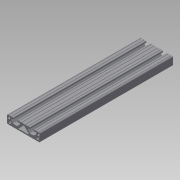
# Autodesk Inventor part: 3034-LITE
Saved by Autodesk Inventor 2013 (Build 170138000, 138)
## iProperties
Created: 2014-04-23
Part Number: 3034-LITE
Material: Generic
Document SubType Name: Modeling
Density: 1 g/cm^3
Vendor: 80/20 Inc.
Engineer: Ross Bowman
Designer: Ross Bowman
Catalog Web Link: 8020.net
Company: 80/20 Inc.
Author: Ross Bowman
Keywords: 80/20 , 8020 , T-Slot , Extrusion
Material: 6105-T5 Aluminum
Autodesk Inventor part; units mm, degrees
ref_plane "YZ Plane" through (0, 0, 0) normal (1, 0, 0) x (0, 1, 0)
ref_plane "XZ Plane" through (0, 0, 0) normal (0, 1, 0) x (-1, 0, 0)
ref_plane "XY Plane" through (0, 0, 0) normal (0, 0, 1) x (1, 0, 0)
sketch "Sketch1" plane through (0, 0, 0) normal (0, 0, 1) x (1, 0, 0)
  circle A0 centre (31.75, -3.175) radius 3.3274
  circle A1 centre (-31.75, -3.175) radius 3.3274
  arc A2 (-30.9118, 7.493) -> (-31.1658, 7.747) centre (-31.1658, 7.493) ccw
  line L0 (-30.9118, 2.5957) -> (-30.9118, 7.493)
  arc A3 (-31.1658, 2.3417) -> (-30.9118, 2.5957) centre (-31.1658, 2.5957) ccw
  line L1 (-36.2712, 2.3417) -> (-31.1658, 2.3417)
  arc A4 (-36.5252, 2.5957) -> (-36.2712, 2.3417) centre (-36.2712, 2.5957) ccw
  line L2 (-36.5252, 4.953) -> (-36.5252, 2.5957)
  arc A5 (-33.7312, 7.747) -> (-36.5252, 4.953) centre (-33.7312, 4.953) ccw
  line L3 (-31.1658, 7.747) -> (-33.7312, 7.747)
  arc A6 (30.9118, 2.5957) -> (31.1658, 2.3417) centre (31.1658, 2.5957) ccw
  line L4 (30.9118, 7.493) -> (30.9118, 2.5957)
  arc A7 (31.1658, 7.747) -> (30.9118, 7.493) centre (31.1658, 7.493) ccw
  line L5 (33.7312, 7.747) -> (31.1658, 7.747)
  arc A8 (36.5252, 4.953) -> (33.7312, 7.747) centre (33.7312, 4.953) ccw
  line L6 (36.5252, 2.5957) -> (36.5252, 4.953)
  arc A9 (36.2712, 2.3417) -> (36.5252, 2.5957) centre (36.2712, 2.5957) ccw
  line L7 (31.1658, 2.3417) -> (36.2712, 2.3417)
  arc A10 (0, 6.0555) -> (-2.3585, 5.1274) centre (-0.1132, 2.8826) ccw
  arc A11 (2.3585, 5.1274) -> (0, 6.0555) centre (0.1132, 2.8826) ccw
  line L8 (11.7359, -4.2517) -> (2.3585, 5.1274)
  arc A12 (10.8378, -6.4196) -> (11.7359, -4.2517) centre (10.8378, -5.1496) ccw
  line L9 (-10.8378, -6.4196) -> (10.8378, -6.4196)
  arc A13 (-11.7359, -4.2517) -> (-10.8378, -6.4196) centre (-10.8378, -5.1496) ccw
  line L10 (-2.3585, 5.1274) -> (-11.7359, -4.2517)
  arc A14 (35.2826, -9.525) -> (38.1, -6.7076) centre (35.2826, -6.7076) ccw
  line L11 (38.1, -6.7076) -> (38.1, 6.7076)
  arc A15 (38.1, 6.7076) -> (35.2826, 9.525) centre (35.2826, 6.7076) ccw
  line L12 (35.2826, 9.525) -> (35.224, 9.525)
  arc A16 (33.7, 9.525) -> (35.224, 9.525) centre (34.462, 9.525) ccw
  line L13 (33.7, 9.525) -> (28.5496, 9.525)
  arc A17 (27.0256, 9.525) -> (28.5496, 9.525) centre (27.7876, 9.525) ccw
  line L14 (27.0256, 9.525) -> (24.7127, 9.525)
  arc A18 (24.7127, 9.525) -> (23.114, 7.9263) centre (24.7127, 7.9263) ccw
  line L15 (23.114, 7.9263) -> (23.114, 7.0358)
  arc A19 (23.114, 7.0358) -> (24.6888, 5.461) centre (24.6888, 7.0358) ccw
  line L16 (24.6888, 5.461) -> (25.8225, 5.461)
  arc A20 (25.8225, 5.461) -> (26.0765, 5.715) centre (25.8225, 5.715) ccw
  line L17 (26.0765, 5.715) -> (26.0765, 5.969)
  arc A21 (26.3305, 6.223) -> (26.0765, 5.969) centre (26.3305, 5.969) ccw
  line L18 (26.3305, 6.223) -> (28.5668, 6.223)
  arc A22 (29.337, 5.4528) -> (28.5668, 6.223) centre (28.5668, 5.4528) ccw
  line L19 (29.337, 5.4528) -> (29.337, 3.4005)
  arc A23 (29.077, 2.7726) -> (29.337, 3.4005) centre (28.4489, 3.4005) ccw
  line L20 (29.077, 2.7726) -> (24.9729, -1.3322)
  arc A24 (21.7509, -2.667) -> (24.9729, -1.3322) centre (21.7509, 1.8892) ccw
  line L21 (21.7509, -2.667) -> (16.4293, -2.667)
  arc A25 (13.0704, -1.2755) -> (16.4293, -2.667) centre (16.4293, 2.0828) ccw
  line L22 (13.0704, -1.2755) -> (9.0233, 2.7723)
  arc A26 (8.763, 3.4008) -> (9.0233, 2.7723) centre (9.6519, 3.4008) ccw
  line L23 (8.763, 3.4008) -> (8.763, 5.4528)
  arc A27 (9.5332, 6.223) -> (8.763, 5.4528) centre (9.5332, 5.4528) ccw
  line L24 (9.5332, 6.223) -> (11.7695, 6.223)
  arc A28 (12.0235, 5.969) -> (11.7695, 6.223) centre (11.7695, 5.969) ccw
  line L25 (12.0235, 5.969) -> (12.0235, 5.715)
  arc A29 (12.0235, 5.715) -> (12.2775, 5.461) centre (12.2775, 5.715) ccw
  line L26 (12.2775, 5.461) -> (13.4112, 5.461)
  arc A30 (13.4112, 5.461) -> (14.986, 7.0358) centre (13.4112, 7.0358) ccw
  line L27 (14.986, 7.0358) -> (14.986, 7.9502)
  arc A31 (14.986, 7.9502) -> (13.4112, 9.525) centre (13.4112, 7.9502) ccw
  line L28 (13.4112, 9.525) -> (11.3174, 9.525)
  arc A32 (9.7934, 9.525) -> (11.3174, 9.525) centre (10.5554, 9.525) ccw
  line L29 (9.7934, 9.525) -> (4.7999, 9.525)
  arc A33 (3.2759, 9.525) -> (4.7999, 9.525) centre (4.0379, 9.525) ccw
  line L30 (3.2759, 9.525) -> (-3.2759, 9.525)
  arc A34 (-4.7999, 9.525) -> (-3.2759, 9.525) centre (-4.0379, 9.525) ccw
  line L31 (-4.7999, 9.525) -> (-9.7934, 9.525)
  arc A35 (-11.3174, 9.525) -> (-9.7934, 9.525) centre (-10.5554, 9.525) ccw
  line L32 (-11.3174, 9.525) -> (-13.4112, 9.525)
  arc A36 (-13.4112, 9.525) -> (-14.986, 7.9502) centre (-13.4112, 7.9502) ccw
  line L33 (-14.986, 7.9502) -> (-14.986, 7.0358)
  arc A37 (-14.986, 7.0358) -> (-13.4112, 5.461) centre (-13.4112, 7.0358) ccw
  line L34 (-13.4112, 5.461) -> (-12.2775, 5.461)
  arc A38 (-12.2775, 5.461) -> (-12.0235, 5.715) centre (-12.2775, 5.715) ccw
  line L35 (-12.0235, 5.715) -> (-12.0235, 5.969)
  arc A39 (-11.7695, 6.223) -> (-12.0235, 5.969) centre (-11.7695, 5.969) ccw
  line L36 (-11.7695, 6.223) -> (-9.5332, 6.223)
  arc A40 (-8.763, 5.4528) -> (-9.5332, 6.223) centre (-9.5332, 5.4528) ccw
  line L37 (-8.763, 5.4528) -> (-8.763, 3.4008)
  arc A41 (-9.0233, 2.7723) -> (-8.763, 3.4008) centre (-9.6519, 3.4008) ccw
  line L38 (-9.0233, 2.7723) -> (-13.0704, -1.2755)
  arc A42 (-16.4293, -2.667) -> (-13.0704, -1.2755) centre (-16.4293, 2.0828) ccw
  line L39 (-16.4293, -2.667) -> (-21.7509, -2.667)
  arc A43 (-24.9729, -1.3322) -> (-21.7509, -2.667) centre (-21.7509, 1.8892) ccw
  line L40 (-24.9729, -1.3322) -> (-29.077, 2.7726)
  arc A44 (-29.337, 3.4005) -> (-29.077, 2.7726) centre (-28.4489, 3.4005) ccw
  line L41 (-29.337, 3.4005) -> (-29.337, 5.4528)
  arc A45 (-28.5668, 6.223) -> (-29.337, 5.4528) centre (-28.5668, 5.4528) ccw
  line L42 (-28.5668, 6.223) -> (-26.3305, 6.223)
  arc A46 (-26.0765, 5.969) -> (-26.3305, 6.223) centre (-26.3305, 5.969) ccw
  line L43 (-26.0765, 5.969) -> (-26.0765, 5.715)
  arc A47 (-26.0765, 5.715) -> (-25.8225, 5.461) centre (-25.8225, 5.715) ccw
  line L44 (-25.8225, 5.461) -> (-24.6888, 5.461)
  arc A48 (-24.6888, 5.461) -> (-23.114, 7.0358) centre (-24.6888, 7.0358) ccw
  line L45 (-23.114, 7.0358) -> (-23.114, 7.9263)
  arc A49 (-23.114, 7.9263) -> (-24.7127, 9.525) centre (-24.7127, 7.9263) ccw
  line L46 (-24.7127, 9.525) -> (-27.0256, 9.525)
  arc A50 (-28.5496, 9.525) -> (-27.0256, 9.525) centre (-27.7876, 9.525) ccw
  line L47 (-28.5496, 9.525) -> (-33.7, 9.525)
  arc A51 (-35.224, 9.525) -> (-33.7, 9.525) centre (-34.462, 9.525) ccw
  line L48 (-35.224, 9.525) -> (-35.2826, 9.525)
  arc A52 (-35.2826, 9.525) -> (-38.1, 6.7076) centre (-35.2826, 6.7076) ccw
  line L49 (-38.1, 6.7076) -> (-38.1, -6.7076)
  arc A53 (-38.1, -6.7076) -> (-35.2826, -9.525) centre (-35.2826, -6.7076) ccw
  line L50 (-35.2826, -9.525) -> (-35.224, -9.525)
  arc A54 (-33.7, -9.525) -> (-35.224, -9.525) centre (-34.462, -9.525) ccw
  line L51 (-33.7, -9.525) -> (-28.5496, -9.525)
  arc A55 (-27.0256, -9.525) -> (-28.5496, -9.525) centre (-27.7876, -9.525) ccw
  line L52 (-27.0256, -9.525) -> (-11.0744, -9.525)
  arc A56 (-9.5504, -9.525) -> (-11.0744, -9.525) centre (-10.3124, -9.525) ccw
  line L53 (-9.5504, -9.525) -> (-4.7253, -9.525)
  arc A57 (-3.2013, -9.525) -> (-4.7253, -9.525) centre (-3.9633, -9.525) ccw
  line L54 (-3.2013, -9.525) -> (3.2013, -9.525)
  arc A58 (4.7253, -9.525) -> (3.2013, -9.525) centre (3.9633, -9.525) ccw
  line L55 (4.7253, -9.525) -> (9.5504, -9.525)
  arc A59 (11.0744, -9.525) -> (9.5504, -9.525) centre (10.3124, -9.525) ccw
  line L56 (11.0744, -9.525) -> (27.0256, -9.525)
  arc A60 (28.5496, -9.525) -> (27.0256, -9.525) centre (27.7876, -9.525) ccw
  line L57 (28.5496, -9.525) -> (33.7, -9.525)
  arc A61 (35.224, -9.525) -> (33.7, -9.525) centre (34.462, -9.525) ccw
  line L58 (35.224, -9.525) -> (35.2826, -9.525)
  point P0 (0, 0)
  constraints: 120 point on circle, 118 end point, 62 centre point
extrude "Extrusion1" add sketch "Sketch1" against normal blind 304.8
body "Solid1"
